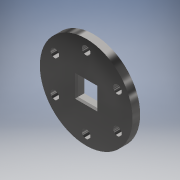
# Autodesk Inventor part: Adam's Shaft plate rev 2
Saved by Autodesk Inventor 2019 (Build 230136000, 136)
## iProperties
Created: 2018-11-07
Part Number: Adam's Shaft plate rev 2
Material: Generic
Document SubType Name: Modeling
Designer: robinsat
Density: 1 g/cm^3
Appearance: Steel - Polished
Author: robinsat
Autodesk Inventor part; units mm, degrees
ref_plane "YZ Plane" through (0, 0, 0) normal (1, 0, 0) x (0, 1, 0)
ref_plane "XZ Plane" through (0, 0, 0) normal (0, 1, 0) x (-1, 0, 0)
ref_plane "XY Plane" through (0, 0, 0) normal (0, 0, 1) x (1, 0, 0)
sketch "Sketch1" plane through (0, 0, 0) normal (0, 0, 1) x (1, 0, 0)
  circle A0 centre (0, 0) radius 48.006
  dimension "d0" = 96.012
  constraints: 1 centre point, 1 coincident
  measures "d0" diameter of A0
extrude "Extrusion1" add sketch "Sketch1" along normal blind 7.9375
sketch "Sketch2" plane through (0, 0, 7.9375) normal (0, 0, 1) x (1, 0, 0)
  circle A0 centre (0, 37.5) radius 4.4196
  circle A1 centre (-32.476, 18.75) radius 4.4196
  circle A2 centre (-32.476, -18.75) radius 4.4196
  circle A3 centre (0, -37.5) radius 4.4196
  circle A4 centre (32.476, -18.75) radius 4.4196
  circle A5 centre (32.476, 18.75) radius 4.4196
  circle A6 centre (0, 0) radius 37.5
  dimension "d17" = 75
  dimension "d3" = 8.8392
  dimension "d7" = 360
  constraints: 6 centre point, 2 vertical alignment, 1 coincident, 15 other
  measures "d3" diameter of A0
extrude "Extrusion2" cut sketch "Sketch2" against normal through all contours A0 A6 | A6 A0 | A6 A1 | A1 A6 | A6 A5 | A5 A6 | A6 A2 | A2 A6 | A6 A4 | A4 A6 | A6 A3 | A3 A6
sketch "Sketch3" plane through (0, 0, 7.9375) normal (0, 0, 1) x (1, 0, 0)
  line L0 (-9.9695, -9.9695) -> (9.9695, -9.9695)
  line L1 (9.9695, -9.9695) -> (9.9695, 9.9695)
  line L2 (9.9695, 9.9695) -> (-9.9695, 9.9695)
  line L3 (-9.9695, 9.9695) -> (-9.9695, -9.9695)
  line L4 (-9.9695, -9.9695) -> (9.9695, 9.9695) construction
  line L5 (9.9695, -9.9695) -> (-9.9695, 9.9695) construction
  point P0 (0, 0)
  dimension "d11" = 19.939
  constraints: 12 end point, 2 midpoint, 2 parallel, 2 perpendicular, 1 horizontal
  measures "d11" distance of L1.end L2.end
extrude "Extrusion3" cut sketch "Sketch3" against normal through all
chamfer "Chamfer1" distance 1.5875 angle 45 4 edges at (0, 9.9695, 7.9375) (-9.9695, 0, 7.9375) (0, -9.9695, 7.9375) (9.9695, 0, 7.9375)
body "Solid1"
